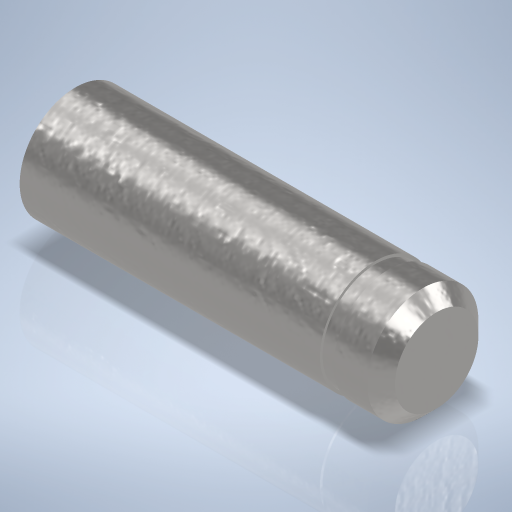
# Autodesk Inventor part: Kurbelzapfen
Saved by Autodesk Inventor 2024 (Build 280153000, 153)
## iProperties
Created: 2024-01-15
Part Number: Kurbelzapfen
Material: Stahl, galvanisiert
Document SubType Name: Modeling
Designer: ffogue
Density: 7.85 g/cm^3
Appearance: Galvanisiert
Author: ffogue
Autodesk Inventor part; units mm, degrees
ref_plane "YZ Plane" through (0, 0, 0) normal (1, 0, 0) x (0, 1, 0)
ref_plane "XZ Plane" through (0, 0, 0) normal (0, 1, 0) x (-1, 0, 0)
ref_plane "XY Plane" through (0, 0, 0) normal (0, 0, 1) x (1, 0, 0)
sketch "Skizze1" plane through (0, 0, 0) normal (0, 0, 1) x (1, 0, 0)
  line L0 (0, 0) -> (0, 2)
  line L1 (0, 2) -> (10.8, 2)
  line L2 (10.8, 2) -> (10.8, 1.9)
  line L3 (10.8, 1.9) -> (11.3, 1.9)
  line L4 (11.3, 1.9) -> (11.3, 2)
  line L5 (11.3, 2) -> (13, 2)
  line L6 (13, 2) -> (13, 0)
  line L7 (0, 0) -> (13, 0)
  point P0 (10.8, 1.95)
  point P1 (0, 1)
  dimension "d0" = 13
  dimension "d1" = 0.5
  dimension "d2" = 10.8
  dimension "d4" = 3.8
  dimension "d5" = 4
  constraints: 16 end point, 5 perpendicular, 2 midpoint, 2 point on line, 1 coincident, 1 horizontal, 1 vertical
  measures "d0" distance of L0.start L6.end
  measures "d1" distance of L3.end L2.end
  measures "d2" horizontal distance of point (10.8, 1.95) point (0, 1)
  measures "d4" diameter of L3.end L7
  measures "d5" diameter of L1 L7
revolve "Umdrehung1" add sketch "Skizze1" angle 360 about axis through (0, 0, 0) along (1, 0, 0)
chamfer "Fasen1" distance 0.5 angle 45 1 edges at (13, -2, 0)
